Autodesk Fusion 360 part; units mm, degrees
note: some values were not read from the file. Chosen so that the rebuilt part matches the saved one: which face or edge a step refers to; which bodies a step acts on; which pieces of a blend or face edit are solid. Set by a fixed rule: which sketch regions a step uses.
(part 2 of 2)
sketch "Sketch34" plane through (0, 0, 158.75) normal (0, 0, -1) x (1, 0, 0)
  line L0 (-5.7308, 8.2) -> (-5.7308, 8.1923)
  line L1 (-5.7308, 8.1923) -> (-5.7765, 3.7202)
  line L2 (-5.7765, 3.7202) -> (-8.3951, 3.7202)
  line L3 (-8.3951, 3.7202) -> (-8.3951, 8.2)
  line L4 (-8.3951, 8.2) -> (-9.937, 8.2)
  line L5 (-9.937, 8.2) -> (-9.937, -7)
  line L6 (-9.937, -7) -> (11.8701, -7)
  line L7 (11.8701, -7) -> (11.8701, -9.1894)
  line L8 (11.8701, -9.1894) -> (31.2057, -10.7944)
  spline S0 degree 5 poles (31.2057, -10.7944) (31.3407, -10.3619) (31.5987, -9.4971) (31.9499, -8.2001) (32.3455, -6.4712) (32.7107, -4.311) (32.9348, -2.1517) (33.0065, 0.0065) (32.9195, 2.1636) (32.6799, 4.3197) (32.2993, 6.4748) (31.8912, 8.1982) (31.5306, 9.4904) (31.2664, 10.3517) (31.1283, 10.7823) knots 0 0 0 0 0 0 0.1 0.2 0.3 0.4 0.5 0.6 0.7 0.8 0.9 1 1 1 1 1 1
  line L9 (31.1283, 10.7823) -> (-0.0496, 8.2)
  line L10 (-0.0496, 8.2) -> (-5.7308, 8.2)
  circle A0 centre (28.0642, 7.769) radius 0.75
  circle A1 centre (28.0642, -5.731) radius 0.75
  line L11 (7.9392, -2.356) -> (7.9392, -5.106)
  line L12 (7.9392, -5.106) -> (3.1892, -5.106)
  line L13 (3.1892, -5.106) -> (3.1892, -2.356)
  line L14 (3.1892, -2.356) -> (7.9392, -2.356)
  line L15 (-4.5429, 7) -> (-4.5887, 2.5202)
  line L16 (-4.5887, 2.5202) -> (-8.737, 2.5202)
  line L17 (-8.737, 2.5202) -> (-8.737, -5.8)
  line L18 (-8.737, -5.8) -> (13.0701, -5.8)
  line L19 (13.0701, -5.8) -> (13.0701, -8.0849)
  line L20 (13.0701, -8.0849) -> (30.3359, -9.5181)
  spline S1 degree 3 poles (30.3359, -9.5181) (31.4433, -5.6729) (31.9621, -1.8721) (31.6959, 1.9204) (31.5194, 4.4349) (31.0197, 6.966) (30.2662, 9.5068) knots 0.043671 0.043671 0.043671 0.043671 0.592631 0.592631 0.592631 0.956608 0.956608 0.956608 0.956608
  line L21 (30.2662, 9.5068) -> (0, 7)
  line L22 (0, 7) -> (-4.5429, 7)
  spline S2 degree 3 poles (30.2992, -9.4648) (31.3914, -5.6585) (31.9058, -1.897) (31.6503, 1.8553) (31.4789, 4.3731) (30.982, 6.9081) (30.2298, 9.4536) knots 0.045546 0.045546 0.045546 0.045546 0.589654 0.589654 0.589654 0.954745 0.954745 0.954745 0.954745
  line L23 (30.2298, 9.4536) -> (0.0021, 6.95)
  line L24 (0.0021, 6.95) -> (-4.4934, 6.95)
  line L25 (-4.4934, 6.95) -> (-4.5392, 2.4702)
  line L26 (-4.5392, 2.4702) -> (-8.687, 2.4702)
  line L27 (-8.687, 2.4702) -> (-8.687, -5.75)
  line L28 (-8.687, -5.75) -> (13.1201, -5.75)
  line L29 (13.1201, -5.75) -> (13.1201, -8.0389)
  line L30 (13.1201, -8.0389) -> (30.2992, -9.4648)
  line L31 (19.0755, -8.5332) -> (19.0755, 8.5297)
  line L32 (24.3447, -9.0208) -> (24.3447, 9.0163)
  line L33 (19.0755, -7.3291) -> (24.3447, -7.7665)
  line L34 (19.0755, 7.3256) -> (24.3447, 7.7621)
  line L35 (24.3057, 11.4715) -> (19.0365, 11.0351)
  line L36 (24.3057, 11.4715) -> (24.3057, 10.2172)
  line L37 (19.0365, 11.0351) -> (19.0365, 9.7808)
  line L38 (24.3057, 10.2674) -> (19.0365, 9.831)
  dimension "d195" = -1.2
  dimension "d196" = -1.25
  dimension "d197" = 1.2
  dimension "d198" = 1.2
  dimension "d201" = 1.25
  dimension "d202" = 0.05
  constraint coincident L30 L31.start
  constraint coincident L23 L31.end
  constraint vertical L31
  constraint coincident L20 L32.start
  constraint coincident L21 L32.end
  constraint parallel L31 L32
  constraint coincident L31 L33.start
  constraint coincident L32 L33.end
  constraint parallel L30 L33
  constraint coincident L31 L34.start
  constraint coincident L32 L34.end
  constraint parallel L23 L34
  constraint parallel L9 L35
  constraint coincident L9 L36.end
  constraint parallel L32 L36
  constraint coincident L9 L37.end
  constraint parallel L36 L37
  constraint coincident L36 L38.start
  constraint coincident L37 L38.end
  constraint parallel L9 L38
  measures "d197" distance of L23 L34
  measures "d198" distance of L30 L33
  measures "d201" distance of L9 L35
  measures "d202" distance of L9 L38
extrude "Extrude43" add sketch "Sketch34" along normal blind 5 contours L23 L31 L32 L34 | L30 L31 L32 L33 bodies 7
extrude "Extrude44" add sketch "Sketch34" against normal blind 1.2 contours L9 L36 L37 L38 | L35 L36 L37 L38 bodies 7
extrude "Extrude45" add sketch "Sketch34" along normal blind 5 contours L35 L36 L37 L38 bodies 7
mirror "Mirror10" about plane through (0, 0, 0) normal (0, 1, 0) of "Extrude44", "Extrude45"
equation "d66 = 45 deg + 22.5 deg"
equation "d67 = 90 deg + 22.5 deg"
equation "d69 = 112.5 deg + 22.5 deg"
equation "d75 = -0.9 mm - 2.2 mm"
named bodies: "Base", "UpperBase", "HoldingDisc", "UnderCap", "Cap", "Support"
